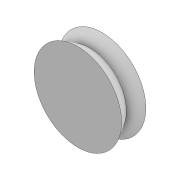
# Autodesk Inventor part: wheel
Saved by Autodesk Inventor 2020 (Build 240168000, 168)
## iProperties
Created: 2020-08-31
Part Number: wheel
Material: 일반
Document SubType Name: Modeling
Designer: 이호석
Mass: 1.0328 g
Surface Area: 8.42609 cm^2
Volume: 1.0328 cm^3
Density: 1 g/cm^3
Appearance: 기본값
Author: 이호석
Autodesk Inventor part; units mm, degrees
ref_plane "YZ Plane" through (0, 0, 0) normal (1, 0, 0) x (0, 1, 0)
sketch "스케치1" plane through (0, 0, 0) normal (0, 0, 1) x (1, 0, 0)
  circle A0 centre (0, 0) radius 9
  dimension "d0" = 18
  constraints: 1 centre point, 1 coincident
  measures "d0" diameter of A0
ref_plane "작업 평면2" through (0, 0, 2.5) normal (0, 0, 1) x (1, 0, 0)
sketch "스케치2" plane through (0, 0, 2.5) normal (0, 0, 1) x (1, 0, 0)
  circle A0 centre (0, 0) radius 7.5
  dimension "d3" = 15
  constraints: 1 centre point, 1 coincident
  measures "d3" diameter of A0
ref_plane "작업 평면1" through (0, 0, 5) normal (0, 0, 1) x (1, 0, 0)
sketch "스케치3" plane through (0, 0, 5) normal (0, 0, 1) x (1, 0, 0)
  circle A0 centre (0, 0) radius 9
  constraints: 1 centre point, 1 coincident
loft "로프트1" add profiles "스케치3", "스케치2"
loft "로프트2" add profiles "스케치1" section 2 edges at (-7.5, 0, 2.5)
sketch "스케치4" plane through (0, 0, 0) normal (0, 0, -1) x (-1, 0, 0)
  circle A0 centre (0, 0) radius 2.5
  dimension "d13" = 5
  constraints: 1 centre point, 1 coincident
  measures "d13" diameter of A0
extrude "돌출2" cut sketch "스케치4" against normal blind 2
